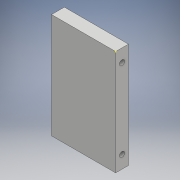
# Autodesk Inventor part: spacermoteur
Saved by Autodesk Inventor 2017 SP1 (Build 210196100, 196)
## iProperties
Part Number: spacermoteur
Material: Générique
Document SubType Name: Modeling
Designer: Sylvain
Density: 1 g/cm^3
Appearance: Par défaut
Author: Sylvain
Autodesk Inventor part; units mm, degrees
ref_plane "YZ Plane" through (0, 0, 0) normal (1, 0, 0) x (0, 1, 0)
ref_plane "XZ Plane" through (0, 0, 0) normal (0, 1, 0) x (-1, 0, 0)
ref_plane "XY Plane" through (0, 0, 0) normal (0, 0, 1) x (1, 0, 0)
sketch "Esquisse1" plane through (0, 0, 0) normal (0, 1, 0) x (-1, 0, 0)
  line L0 (50, 0) -> (0, 0)
  line L1 (0, 0) -> (0, -82)
  line L2 (0, -82) -> (50, -82)
  line L3 (50, -82) -> (50, 0)
  point P0 (0, 0)
  dimension "d0" = 0
  dimension "d1" = 0
  dimension "d2" = 50
  dimension "d3" = 82
  constraints: 8 end point, 2 parallel, 1 horizontal, 1 perpendicular
  measures "d0" distance from line of point (0, 0) L0
  measures "d1" distance from line of point (0, 0) L1
  measures "d2" distance between parallel lines of L1 L3
  measures "d3" distance of L2.end L0.start
extrude "Extrusion1" add sketch "Esquisse1" along normal blind 10
sketch "Esquisse2" plane through (-50, 0, 0) normal (0, 0, 1) x (1, 0, 0)
  point P0 (50, 0)
sketch "Esquisse3" plane through (0, 0, 0) normal (1, 0, 0) x (0, 0, -1)
  line L0 (10, 5) -> (72, 5)
  line L1 (0, 0) -> (0, 10) projected
  circle A0 centre (10, 5) radius 2
  circle A1 centre (72, 5) radius 2
  line L2 (0, 10) -> (82, 10) projected
  dimension "d7" = 62
  dimension "d8" = 10
  dimension "d9" = 4
  dimension "d10" = 4
  dimension "d11" = 5
  constraints: 2 centre point, 2 coincident, 2 end point, 1 horizontal
  measures "d7" distance of L0.start L0.end
  measures "d8" distance from line of L1 L0.start
  measures "d9" diameter of A0
  measures "d10" diameter of A1
  measures "d11" distance between parallel lines of L2 L0
hole "Perçage1" at (0, 5, -10) at (0, 5, -72) direction (-1, 0, 0) diameter 4 end through all
